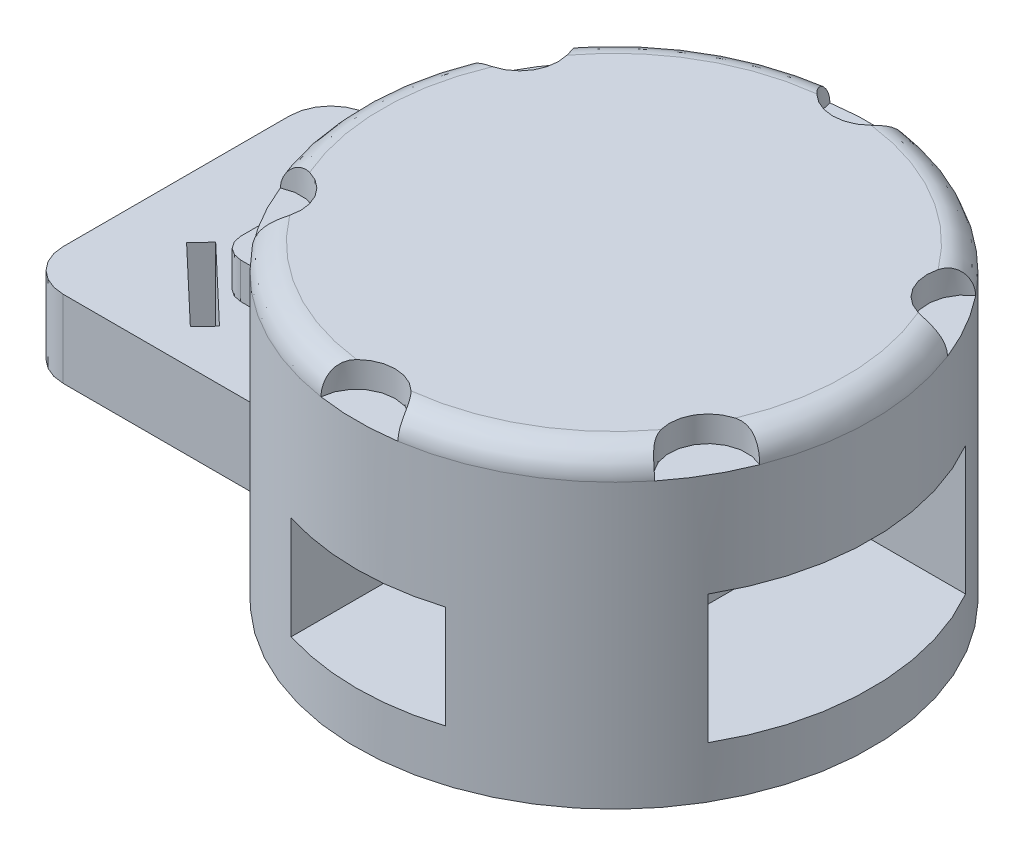
# Autodesk Inventor part: redondogas
Saved by Autodesk Inventor 2015 (Build 190159000, 159)
## iProperties
Created: 2017-09-28
Part Number: redondogas
Material: Generic
Document SubType Name: Modeling
Designer: Max
Density: 1 g/cm^3
Appearance: Default
Author: Max
Autodesk Inventor part; units mm, degrees
sketch "Sketch1" plane through (0, 0, 0) normal (0, 1, 0) x (-1, 0, 0)
  circle A0 centre (0, 0) radius 50
  dimension "d0" = 100
  constraints: 1 centre point, 1 coincident
  measures "d0" diameter of A0
extrude "Extrusion1" add sketch "Sketch1" along normal blind 60
sketch "Sketch2" plane through (0, 60, 0) normal (0, 1, 0) x (1, 0, 0)
  circle A0 centre (0, 0) radius 50 projected
  circle A1 centre (0, 50) radius 7.5
  circle A2 centre (43.3013, 25) radius 7.5
  circle A3 centre (43.3013, -25) radius 7.5
  circle A4 centre (0, -50) radius 7.5
  circle A5 centre (-43.3013, -25) radius 7.5
  circle A6 centre (-43.3013, 25) radius 7.5
  dimension "d3" = 15
  dimension "d6" = 360
  constraints: 6 centre point, 2 coincident, 1 vertical alignment, 23 other
  measures "d3" diameter of A1
fillet "Fillet1" radius 5 1 edges at (50, 60, 0)
extrude "Extrusion2" cut sketch "Sketch2" against normal blind 5 contours A2 A0 | A0 A2 | A3 A0 | A0 A3 | A1 A0 | A0 A1 | A4 A0 | A0 A4 | A6 A0 | A0 A6 | A5 A0 | A0 A5
ref_plane "Work Plane1" through (-50, 55, 0) normal (-1, 0, 0) x (0, -1, 0)
sketch "Sketch4" plane through (-50, 55, 0) normal (-1, 0, 0) x (0, -1, 0)
  line L0 (27.2118, -30) -> (42.2118, -30)
  line L1 (42.2118, -30) -> (42.2118, 30)
  line L2 (42.2118, 30) -> (27.2118, 30)
  line L3 (27.2118, 30) -> (27.2118, -30)
  point P0 (55, 0)
  dimension "d14" = 60
  dimension "d15" = 15
  constraints: 8 end point, 2 parallel, 1 horizontal, 1 perpendicular
  measures "d14" distance of L1.end L0.end
  measures "d15" distance between parallel lines of L1 L3
extrude "Extrusion4" add sketch "Sketch4" along normal mid plane 70
sketch "Sketch5" plane through (-50, 55, 0) normal (-1, 0, 0) x (0, -1, 0)
  line L0 (27.2118, 30) -> (27.2118, -30) projected
  line L1 (27.2118, 14) -> (20.2118, 14)
  line L2 (20.2118, 14) -> (20.2118, -14)
  line L3 (20.2118, -14) -> (27.2118, -14)
  line L4 (27.2118, -14) -> (27.2118, 14)
  point P0 (55, 0)
  dimension "d18" = 7
  dimension "d19" = 28
  constraints: 8 end point, 2 parallel, 1 horizontal, 1 perpendicular, 1 point on line
  measures "d18" distance of L3.end L2.end
  measures "d19" distance of L2.end L1.end
extrude "Extrusion5" add sketch "Sketch5" along normal mid plane 25
fillet "Fillet2" radius 8 2 edges at (-85, 20.2882, -30) (-85, 20.2882, 30)
sketch "Sketch6" plane through (-62.5, 27.7882, 14) normal (0, 1, 0) x (1, 0, 0)
  point P0 (62.5, 14)
ref_plane "Work Plane2" through (-62.5, 34.7882, 0) normal (0, 1, 0) x (1, 0, 0)
sketch "Sketch7" plane through (-62.5, 34.7882, 0) normal (0, 1, 0) x (1, 0, 0)
  line L0 (6.0723, 20.1953) -> (-8.4303, 6.4231)
  line L1 (-8.4303, 6.4231) -> (-11.1847, 9.3236)
  line L2 (-11.1847, 9.3236) -> (3.3179, 23.0958)
  line L3 (3.3179, 23.0958) -> (6.0723, 20.1953)
  line L4 (11.5119, 0) -> (-21.1929, 0)
  line L5 (6.0723, -20.1953) -> (-8.4303, -6.4231)
  line L6 (-8.4303, -6.4231) -> (-11.1847, -9.3236)
  line L7 (-11.1847, -9.3236) -> (3.3179, -23.0958)
  line L8 (3.3179, -23.0958) -> (6.0723, -20.1953)
  point P0 (62.5, 0)
  dimension "d23" = 20
  dimension "d24" = 4
  constraints: 18 end point, 4 symmetric about line, 3 perpendicular, 1 horizontal
  measures "d23" distance of L0.start L0.end
  measures "d24" distance of L0.end L1.end
extrude "Extrusion6" cut sketch "Sketch7" against normal blind 50
fillet "Fillet3" radius 4 2 edges at (-62.5, 31.2882, -14) (-62.5, 31.2882, 14)
sketch "Sketch11" plane through (0, 0, 0) normal (0, 0, 1) x (1, 0, 0)
  line L0 (-15, 10) -> (15, 10)
  line L1 (15, 10) -> (15, 30)
  line L2 (15, 30) -> (-15, 30)
  line L3 (-15, 30) -> (-15, 10)
  point P0 (0, 0)
  dimension "d29" = 30
  dimension "d30" = 20
  constraints: 8 end point, 2 parallel, 1 horizontal, 1 perpendicular
  measures "d29" distance of L2.end L1.end
  measures "d30" distance of L1.end L0.end
extrude "Extrusion7" cut sketch "Sketch11" along normal mid plane 100
sketch "Sketch12" plane through (0, 0, 0) normal (0, 0, 1) x (1, 0, 0)
  line L0 (-15, 10) -> (15, 10)
  line L1 (15, 10) -> (15, 30)
  line L2 (15, 30) -> (-15, 30)
  line L3 (-15, 30) -> (-15, 10)
  point P0 (0, 0)
  dimension "d33" = 30
  dimension "d34" = 20
  constraints: 8 end point, 2 parallel, 1 horizontal, 1 perpendicular
  measures "d33" distance of L2.end L1.end
  measures "d34" distance of L1.end L0.end
extrude "Extrusion8" add sketch "Sketch12" along normal mid plane 40
ref_plane "Work Plane7" through (22.6604, 3.5721, 0) normal (-0.766, 0.6428, 0) x (0, 0, 1)
ref_plane "Work Plane6" through (15, 10, 0) normal (-0.766, 0.6428, 0) x (0, 0, 1)
ref_plane "Work Plane8" through (20, 0, 0) normal (1, 0, 0) x (0, 1, 0)
sketch "Sketch18" plane through (20, 0, 0) normal (1, 0, 0) x (0, 1, 0)
  line L0 (10, 25) -> (35, 25)
  line L1 (35, 25) -> (35, -25)
  line L2 (35, -25) -> (10, -25)
  line L3 (10, -25) -> (10, 25)
  dimension "d52" = 25
  dimension "d53" = 50
  constraints: 8 end point, 2 parallel, 1 horizontal, 1 perpendicular
  measures "d52" distance of L1.end L2.end
  measures "d53" distance of L0.end L1.end
extrude "Extrusion11" cut sketch "Sketch18" along normal blind 30
body "Solid1"
